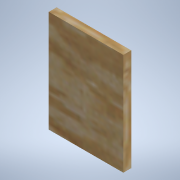
# Autodesk Inventor part: Side slant
Saved by Autodesk Inventor 2020 (Build 240168000, 168)
## iProperties
Created: 2020-01-25
Part Number: Side slant
Material: Wood (Oak)
Document SubType Name: Modeling
Designer: 1cikaychapman
Density: 0.76 g/cm^3
Appearance: Plywood - Weathered
Author: 1cikaychapman
Autodesk Inventor part; units mm, degrees
ref_plane "YZ Plane" through (0, 0, 0) normal (1, 0, 0) x (0, 1, 0)
ref_plane "XZ Plane" through (0, 0, 0) normal (0, 1, 0) x (-1, 0, 0)
ref_plane "XY Plane" through (0, 0, 0) normal (0, 0, 1) x (1, 0, 0)
sketch "Sketch1" plane through (0, 0, 0) normal (0, 0, 1) x (1, 0, 0)
  line L0 (0, 0) -> (120.65, 0)
  line L1 (120.65, 0) -> (120.65, 165.1)
  line L2 (120.65, 165.1) -> (0, 165.1)
  line L3 (0, 165.1) -> (0, 0)
  dimension "d0" = 120.65
  dimension "d1" = 165.1
  constraints: 8 end point, 2 parallel, 1 horizontal, 1 perpendicular
  measures "d0" distance of L2.end L1.end
  measures "d1" distance of L1.end L0.end
extrude "Extrusion1" add sketch "Sketch1" along normal blind 12.7
body "Solid1"
